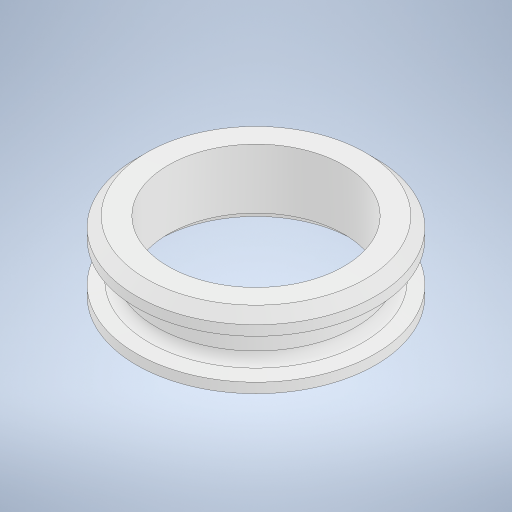
# Autodesk Inventor part: Weapon Pulley
Saved by Autodesk Inventor 2023.2 (Build 272271000, 271)
## iProperties
Created: 2023-04-13
Part Number: Weapon Pulley
Material: UHMW, White
Document SubType Name: Modeling
Designer: Nathan Cai
Density: 0.94 g/cm^3
Appearance: Smooth - White
Mass: 3.78057 g
Surface Area: 36.616 cm^2
Volume: 4.02188 cm^3
Author: Nathan Cai
Autodesk Inventor part; units mm, degrees
ref_plane "YZ Plane" through (0, 0, 0) normal (1, 0, 0) x (0, 1, 0)
ref_plane "XZ Plane" through (0, 0, 0) normal (0, 1, 0) x (-1, 0, 0)
ref_plane "XY Plane" through (0, 0, 0) normal (0, 0, 1) x (1, 0, 0)
sketch "Sketch1" plane through (0, 0, 0) normal (0, 0, 1) x (1, 0, 0)
  line L0 (0, 0) -> (14, 0) construction
  line L1 (14, 0) -> (14, 12.7)
  line L2 (14, 12.7) -> (0, 12.7) construction
  line L3 (0, 12.7) -> (0, 0) construction
  line L4 (14, 6.35) -> (19.05, 6.35) construction
  line L5 (15.875, 3.175) -> (19.05, 3.175) construction
  line L6 (19.05, 3.175) -> (19.05, 9.525) construction
  line L7 (19.05, 9.525) -> (15.875, 9.525) construction
  line L8 (15.875, 9.525) -> (15.875, 3.175)
  line L9 (15.875, 3.175) -> (19.05, 9.525) construction
  line L10 (19.05, 3.175) -> (15.875, 9.525) construction
  line L11 (19.05, 9.525) -> (15.875, 8.6743)
  line L12 (19.05, 3.175) -> (15.875, 4.0257)
  line L13 (15.875, 0) -> (19.05, 0) construction
  line L14 (19.05, 0) -> (19.05, 12.7)
  line L15 (19.05, 12.7) -> (15.875, 12.7) construction
  line L16 (15.875, 12.7) -> (15.875, 0) construction
  line L17 (15.875, 0) -> (19.05, 12.7) construction
  line L18 (19.05, 0) -> (15.875, 12.7) construction
  line L19 (14, 12.7) -> (19.05, 12.7)
  line L20 (14, 0) -> (19.05, 0)
  line L21 (19.05, 1.5875) -> (14, 1.5875)
  point P0 (17.4625, 6.35)
  point P1 (19.05, 3.175)
  point P2 (15.875, 4.0257)
  point P3 (19.05, 9.525)
  dimension "d0" = 14
  dimension "d1" = 12.7
  dimension "d3" = 6.35
  dimension "d4" = 3.175
  dimension "d5" = 15
  dimension "d6" = 3.175
  dimension "d7" = 12.7
  dimension "d16" = 19.05
  dimension "d17" = 1.5875
  constraints: 44 end point, 7 parallel, 6 midpoint, 4 perpendicular, 4 point on line, 3 horizontal, 1 symmetric about line
  measures "d0" distance of L2.end L1.end
  measures "d1" distance of L1.end L0.end
  measures "d3" distance of L6.end L5.end
  measures "d4" distance between parallel lines of L6 L8
  measures "d5" angle of L4 L11
  measures "d6" distance of L15.end L14.end
  measures "d7" distance of L14.end L13.end
  measures "d16" distance between parallel lines of L3 L14
  measures "d17" distance between parallel lines of L13 L21
revolve "Revolution1" add sketch "Sketch1" angle 360 about axis through (0, 12.7, 0) along (0, -1, 0) contours L1 L19 L14 L11 L8 L12 L21
chamfer "Chamfer1" distance 1.5875 angle 45 1 edges at (-19.05, 12.7, 0)
fillet "Fillet1" radius 1.5875 2 edges at (-15.875, 8.6743, 0) (-15.875, 4.0257, 0)
chamfer "Chamfer3" distance 1.5875 angle 45 1 edges at (-14, 1.5875, 0)
equation "\"d6\" = d4"
body "Solid1"
